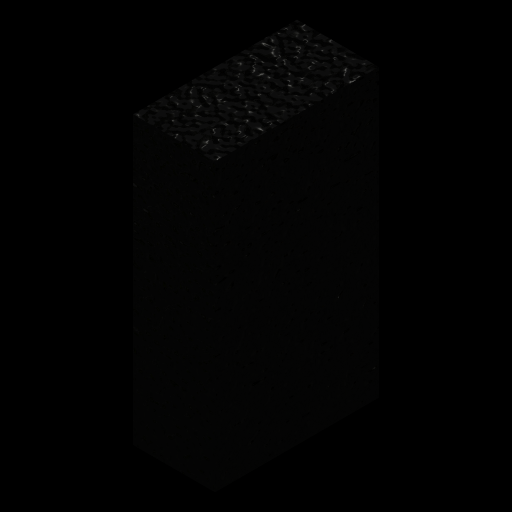
# Autodesk Inventor part: BatteryPlaceholder
Saved by Autodesk Inventor 2023 (Build 270158030, 158C)
## iProperties
Created: 2022-11-17
Part Number: BatteryPlaceholder
Material: Air
Document SubType Name: Modeling
Designer: kumpu
Density: 0.0012 g/cm^3
Appearance: Black
Author: kumpu
Autodesk Inventor part; units mm, degrees
ref_plane "YZ Plane" through (0, 0, 0) normal (1, 0, 0) x (0, 1, 0)
ref_plane "XZ Plane" through (0, 0, 0) normal (0, 1, 0) x (-1, 0, 0)
ref_plane "XY Plane" through (0, 0, 0) normal (0, 0, 1) x (1, 0, 0)
sketch "Sketch1" plane through (0, 0, 0) normal (0, 1, 0) x (-1, 0, 0)
  line L0 (39.5, 79) -> (-39.5, 79)
  line L1 (-39.5, 79) -> (-39.5, -79)
  line L2 (-39.5, -79) -> (39.5, -79)
  line L3 (39.5, -79) -> (39.5, 79)
  line L4 (39.5, 79) -> (-39.5, -79) construction
  line L5 (-39.5, 79) -> (39.5, -79) construction
  point P0 (0, 0)
  dimension "d0" = 158
  dimension "d1" = 79
  constraints: 12 end point, 2 midpoint, 2 parallel, 1 horizontal, 1 perpendicular
  measures "d0" distance of L2.end L0.start
  measures "d1" distance of L1.end L2.end
extrude "Extrusion1" add sketch "Sketch1" along normal blind 276
body "Solid1"
